Autodesk Fusion 360 part; units mm, degrees
(part 2 of 2)
  spline S7 degree 5 poles (3.1969, -8.4131) (3.199, -8.4065) (3.2031, -8.3933) (3.2093, -8.3736) (3.2174, -8.3472) (3.2273, -8.3143) (3.237, -8.2814) (3.2465, -8.2485) (3.2557, -8.2156) (3.2647, -8.1828) (3.2735, -8.1499) (3.282, -8.1171) (3.2903, -8.0843) (3.2983, -8.0515) (3.3062, -8.0188) (3.3138, -7.986) (3.3211, -7.9533) (3.3282, -7.9206) (3.3351, -7.888) (3.3418, -7.8554) (3.3482, -7.8228) (3.3543, -7.7902) (3.3602, -7.7577) (3.3659, -7.7253) (3.3713, -7.6928) (3.3765, -7.6604) (3.3814, -7.6281) (3.3861, -7.5958) (3.3906, -7.5635) (3.3947, -7.5313) (3.3987, -7.4991) (3.4023, -7.467) (3.4058, -7.4349) (3.4089, -7.4029) (3.4118, -7.371) (3.4145, -7.3391) (3.4169, -7.3073) (3.419, -7.2755) (3.4208, -7.2438) (3.4224, -7.2122) (3.4238, -7.1806) (3.4248, -7.1491) (3.4256, -7.1177) (3.426, -7.0864) (3.4262, -7.0551) (3.4262, -7.024) (3.4258, -6.9929) (3.4252, -6.9619) (3.4242, -6.931) (3.423, -6.9002) (3.4215, -6.8695) (3.4196, -6.8389) (3.4175, -6.8084) (3.415, -6.778) (3.4121, -6.7477) (3.409, -6.7176) (3.4055, -6.6876) (3.4018, -6.6576) (3.3978, -6.6278) (3.3934, -6.5981) (3.3886, -6.5686) (3.3833, -6.5393) (3.3775, -6.5102) (3.3713, -6.4813) (3.3645, -6.4526) (3.3575, -6.424) (3.3502, -6.3955) (3.3426, -6.3672) (3.3348, -6.339) (3.3263, -6.3112) (3.3168, -6.2838) (3.3081, -6.2623) (3.3008, -6.2466) (3.2955, -6.2363) (3.2928, -6.2312) knots -1 -1 -1 -1 -1 -1 -0.98571429 -0.97142857 -0.95714286 -0.94285714 -0.92857143 -0.91428571 -0.9 -0.88571429 -0.87142857 -0.85714286 -0.84285714 -0.82857143 -0.81428571 -0.8 -0.78571429 -0.77142857 -0.75714286 -0.74285714 -0.72857143 -0.71428571 -0.7 -0.68571429 -0.67142857 -0.65714286 -0.64285714 -0.62857143 -0.61428571 -0.6 -0.58571429 -0.57142857 -0.55714286 -0.54285714 -0.52857143 -0.51428571 -0.5 -0.48571429 -0.47142857 -0.45714286 -0.44285714 -0.42857143 -0.41428571 -0.4 -0.38571429 -0.37142857 -0.35714286 -0.34285714 -0.32857143 -0.31428571 -0.3 -0.28571429 -0.27142857 -0.25714286 -0.24285714 -0.22857143 -0.21428571 -0.2 -0.18571429 -0.17142857 -0.15714286 -0.14285714 -0.12857143 -0.11428571 -0.1 -0.08571429 -0.07142857 -0.05714286 -0.04285714 -0.02857143 -0.01428571 0 0 0 0 0 0
  line L7 (3.2928, -6.2312) -> (2.9176, -5.521)
  arc A15 (3.0915, -4.8654) -> (2.9176, -5.521) centre (3.3596, -5.2874) ccw
  arc A16 (3.0915, -4.8654) -> (3.672, -4.4437) centre (0, 0) ccw
  arc A17 (4.3492, -4.4809) -> (3.672, -4.4437) centre (3.9905, -4.8291) ccw
  line L8 (4.3492, -4.4809) -> (4.9086, -5.0572)
  spline S8 degree 5 poles (4.9086, -5.0572) (4.9127, -5.0613) (4.9209, -5.0695) (4.9336, -5.0813) (4.9513, -5.0962) (4.9744, -5.1137) (4.9983, -5.1304) (5.0226, -5.1466) (5.0473, -5.1625) (5.0721, -5.1783) (5.097, -5.1938) (5.1223, -5.2091) (5.1478, -5.224) (5.1737, -5.2385) (5.2, -5.2525) (5.2266, -5.2662) (5.2535, -5.2796) (5.2806, -5.2926) (5.3079, -5.3054) (5.3354, -5.318) (5.3631, -5.3303) (5.391, -5.3423) (5.4191, -5.3541) (5.4474, -5.3656) (5.476, -5.3768) (5.5047, -5.3878) (5.5336, -5.3984) (5.5627, -5.4089) (5.592, -5.4191) (5.6215, -5.429) (5.6511, -5.4387) (5.6809, -5.4482) (5.7108, -5.4574) (5.7409, -5.4664) (5.7712, -5.4751) (5.8016, -5.4836) (5.8322, -5.4919) (5.8629, -5.4999) (5.8938, -5.5077) (5.9248, -5.5153) (5.9559, -5.5226) (5.9872, -5.5297) (6.0186, -5.5366) (6.0501, -5.5433) (6.0818, -5.5497) (6.1136, -5.5559) (6.1456, -5.5619) (6.1776, -5.5676) (6.2098, -5.5731) (6.2421, -5.5784) (6.2745, -5.5835) (6.307, -5.5884) (6.3397, -5.593) (6.3724, -5.5975) (6.4053, -5.6017) (6.4383, -5.6056) (6.4713, -5.6094) (6.5045, -5.613) (6.5378, -5.6163) (6.5712, -5.6194) (6.6046, -5.6223) (6.6382, -5.625) (6.6719, -5.6274) (6.7056, -5.6297) (6.7395, -5.6317) (6.7734, -5.6335) (6.8075, -5.6351) (6.8416, -5.6365) (6.8758, -5.6377) (6.9101, -5.6386) (6.9444, -5.6394) (6.972, -5.6398) (6.9927, -5.64) (7.0065, -5.6401) (7.0134, -5.6402) knots 0 0 0 0 0 0 0.01428571 0.02857143 0.04285714 0.05714286 0.07142857 0.08571429 0.1 0.11428571 0.12857143 0.14285714 0.15714286 0.17142857 0.18571429 0.2 0.21428571 0.22857143 0.24285714 0.25714286 0.27142857 0.28571429 0.3 0.31428571 0.32857143 0.34285714 0.35714286 0.37142857 0.38571429 0.4 0.41428571 0.42857143 0.44285714 0.45714286 0.47142857 0.48571429 0.5 0.51428571 0.52857143 0.54285714 0.55714286 0.57142857 0.58571429 0.6 0.61428571 0.62857143 0.64285714 0.65714286 0.67142857 0.68571429 0.7 0.71428571 0.72857143 0.74285714 0.75714286 0.77142857 0.78571429 0.8 0.81428571 0.82857143 0.84285714 0.85714286 0.87142857 0.88571429 0.9 0.91428571 0.92857143 0.94285714 0.95714286 0.97142857 0.98571429 1 1 1 1 1 1
  arc A18 (7.0134, -5.6402) -> (7.5314, -4.9273) centre (0, 0) ccw
  spline S9 degree 5 poles (7.5314, -4.9273) (7.5292, -4.9207) (7.5249, -4.9076) (7.5182, -4.888) (7.5093, -4.8619) (7.498, -4.8294) (7.4865, -4.7971) (7.4748, -4.765) (7.4629, -4.7329) (7.4509, -4.7011) (7.4387, -4.6693) (7.4263, -4.6378) (7.4137, -4.6064) (7.401, -4.5751) (7.3881, -4.544) (7.375, -4.5131) (7.3617, -4.4823) (7.3482, -4.4516) (7.3346, -4.4212) (7.3208, -4.3909) (7.3068, -4.3608) (7.2927, -4.3308) (7.2784, -4.301) (7.2639, -4.2714) (7.2492, -4.242) (7.2343, -4.2127) (7.2193, -4.1837) (7.2041, -4.1548) (7.1887, -4.1261) (7.1732, -4.0976) (7.1574, -4.0692) (7.1415, -4.0411) (7.1255, -4.0131) (7.1092, -3.9854) (7.0928, -3.9578) (7.0762, -3.9305) (7.0594, -3.9033) (7.0425, -3.8764) (7.0253, -3.8496) (7.008, -3.8231) (6.9905, -3.7968) (6.9729, -3.7707) (6.955, -3.7449) (6.937, -3.7192) (6.9188, -3.6938) (6.9004, -3.6687) (6.8819, -3.6437) (6.8631, -3.619) (6.8442, -3.5946) (6.8251, -3.5704) (6.8058, -3.5464) (6.7863, -3.5227) (6.7667, -3.4993) (6.7468, -3.4763) (6.7267, -3.4534) (6.7064, -3.4309) (6.686, -3.4086) (6.6654, -3.3866) (6.6446, -3.3649) (6.6236, -3.3434) (6.6024, -3.3224) (6.5809, -3.3017) (6.5591, -3.2816) (6.537, -3.2619) (6.5147, -3.2426) (6.4922, -3.2236) (6.4695, -3.2049) (6.4468, -3.1864) (6.4239, -3.1683) (6.4006, -3.1507) (6.3768, -3.1341) (6.3572, -3.1219) (6.342, -3.1135) (6.3317, -3.1082) (6.3265, -3.1056) knots -1 -1 -1 -1 -1 -1 -0.98571429 -0.97142857 -0.95714286 -0.94285714 -0.92857143 -0.91428571 -0.9 -0.88571429 -0.87142857 -0.85714286 -0.84285714 -0.82857143 -0.81428571 -0.8 -0.78571429 -0.77142857 -0.75714286 -0.74285714 -0.72857143 -0.71428571 -0.7 -0.68571429 -0.67142857 -0.65714286 -0.64285714 -0.62857143 -0.61428571 -0.6 -0.58571429 -0.57142857 -0.55714286 -0.54285714 -0.52857143 -0.51428571 -0.5 -0.48571429 -0.47142857 -0.45714286 -0.44285714 -0.42857143 -0.41428571 -0.4 -0.38571429 -0.37142857 -0.35714286 -0.34285714 -0.32857143 -0.31428571 -0.3 -0.28571429 -0.27142857 -0.25714286 -0.24285714 -0.22857143 -0.21428571 -0.2 -0.18571429 -0.17142857 -0.15714286 -0.14285714 -0.12857143 -0.11428571 -0.1 -0.08571429 -0.07142857 -0.05714286 -0.04285714 -0.02857143 -0.01428571 0 0 0 0 0 0
  line L9 (6.3265, -3.1056) -> (5.6055, -2.7517)
  arc A19 (5.3609, -2.1191) -> (5.6055, -2.7517) centre (5.8259, -2.3029) ccw
  arc A20 (5.3609, -2.1191) -> (5.5826, -1.4367) centre (0, 0) ccw
  arc A21 (6.1524, -1.0687) -> (5.5826, -1.4367) centre (6.0668, -1.5613) ccw
  line L10 (6.1524, -1.0687) -> (6.9437, -1.2061)
  spline S10 degree 5 poles (6.9437, -1.2061) (6.9494, -1.2071) (6.9609, -1.2089) (6.9781, -1.211) (7.0011, -1.2127) (7.0301, -1.2132) (7.0593, -1.2127) (7.0885, -1.2115) (7.1178, -1.2099) (7.1471, -1.208) (7.1764, -1.2059) (7.2058, -1.2034) (7.2353, -1.2005) (7.2647, -1.197) (7.2943, -1.1929) (7.3238, -1.1884) (7.3534, -1.1833) (7.383, -1.178) (7.4126, -1.1723) (7.4422, -1.1663) (7.4719, -1.1599) (7.5015, -1.1533) (7.5312, -1.1463) (7.5609, -1.139) (7.5906, -1.1313) (7.6202, -1.1232) (7.6499, -1.1148) (7.6796, -1.1062) (7.7093, -1.0972) (7.7389, -1.0879) (7.7686, -1.0784) (7.7983, -1.0685) (7.8279, -1.0584) (7.8575, -1.048) (7.8872, -1.0372) (7.9168, -1.0262) (7.9464, -1.015) (7.9759, -1.0034) (8.0055, -0.9916) (8.035, -0.9795) (8.0645, -0.9671) (8.094, -0.9545) (8.1235, -0.9416) (8.1529, -0.9284) (8.1823, -0.915) (8.2117, -0.9013) (8.241, -0.8874) (8.2704, -0.8732) (8.2996, -0.8587) (8.3289, -0.844) (8.3581, -0.8291) (8.3873, -0.8139) (8.4164, -0.7985) (8.4455, -0.7828) (8.4746, -0.7669) (8.5036, -0.7508) (8.5325, -0.7344) (8.5615, -0.7177) (8.5903, -0.7009) (8.6192, -0.6838) (8.648, -0.6664) (8.6767, -0.6489) (8.7054, -0.6311) (8.734, -0.613) (8.7626, -0.5948) (8.7911, -0.5763) (8.8196, -0.5576) (8.848, -0.5387) (8.8764, -0.5195) (8.9047, -0.5001) (8.9329, -0.4805) (8.9555, -0.4647) (8.9723, -0.4527) (8.9836, -0.4446) (8.9892, -0.4406) knots 0 0 0 0 0 0 0.01428571 0.02857143 0.04285714 0.05714286 0.07142857 0.08571429 0.1 0.11428571 0.12857143 0.14285714 0.15714286 0.17142857 0.18571429 0.2 0.21428571 0.22857143 0.24285714 0.25714286 0.27142857 0.28571429 0.3 0.31428571 0.32857143 0.34285714 0.35714286 0.37142857 0.38571429 0.4 0.41428571 0.42857143 0.44285714 0.45714286 0.47142857 0.48571429 0.5 0.51428571 0.52857143 0.54285714 0.55714286 0.57142857 0.58571429 0.6 0.61428571 0.62857143 0.64285714 0.65714286 0.67142857 0.68571429 0.7 0.71428571 0.72857143 0.74285714 0.75714286 0.77142857 0.78571429 0.8 0.81428571 0.82857143 0.84285714 0.85714286 0.87142857 0.88571429 0.9 0.91428571 0.92857143 0.94285714 0.95714286 0.97142857 0.98571429 1 1 1 1 1 1
  arc A22 (8.9892, -0.4406) -> (8.9892, 0.4406) centre (0, 0) ccw
  spline S11 degree 5 poles (8.9892, 0.4406) (8.9836, 0.4446) (8.9723, 0.4527) (8.9555, 0.4647) (8.9329, 0.4805) (8.9047, 0.5001) (8.8764, 0.5195) (8.848, 0.5387) (8.8196, 0.5576) (8.7911, 0.5763) (8.7626, 0.5948) (8.734, 0.613) (8.7054, 0.6311) (8.6767, 0.6489) (8.648, 0.6664) (8.6192, 0.6838) (8.5903, 0.7009) (8.5615, 0.7177) (8.5325, 0.7344) (8.5036, 0.7508) (8.4746, 0.7669) (8.4455, 0.7828) (8.4164, 0.7985) (8.3873, 0.8139) (8.3581, 0.8291) (8.3289, 0.844) (8.2996, 0.8587) (8.2704, 0.8732) (8.241, 0.8874) (8.2117, 0.9013) (8.1823, 0.915) (8.1529, 0.9284) (8.1235, 0.9416) (8.094, 0.9545) (8.0645, 0.9671) (8.035, 0.9795) (8.0055, 0.9916) (7.9759, 1.0034) (7.9464, 1.015) (7.9168, 1.0262) (7.8872, 1.0372) (7.8575, 1.048) (7.8279, 1.0584) (7.7983, 1.0685) (7.7686, 1.0784) (7.7389, 1.0879) (7.7093, 1.0972) (7.6796, 1.1062) (7.6499, 1.1148) (7.6202, 1.1232) (7.5906, 1.1313) (7.5609, 1.139) (7.5312, 1.1463) (7.5015, 1.1533) (7.4719, 1.1599) (7.4422, 1.1663) (7.4126, 1.1723) (7.383, 1.178) (7.3534, 1.1833) (7.3238, 1.1884) (7.2943, 1.1929) (7.2647, 1.197) (7.2353, 1.2005) (7.2058, 1.2034) (7.1764, 1.2059) (7.1471, 1.208) (7.1178, 1.2099) (7.0885, 1.2115) (7.0593, 1.2127) (7.0301, 1.2132) (7.0011, 1.2127) (6.9781, 1.211) (6.9609, 1.2089) (6.9494, 1.2071) (6.9437, 1.2061) knots -1 -1 -1 -1 -1 -1 -0.98571429 -0.97142857 -0.95714286 -0.94285714 -0.92857143 -0.91428571 -0.9 -0.88571429 -0.87142857 -0.85714286 -0.84285714 -0.82857143 -0.81428571 -0.8 -0.78571429 -0.77142857 -0.75714286 -0.74285714 -0.72857143 -0.71428571 -0.7 -0.68571429 -0.67142857 -0.65714286 -0.64285714 -0.62857143 -0.61428571 -0.6 -0.58571429 -0.57142857 -0.55714286 -0.54285714 -0.52857143 -0.51428571 -0.5 -0.48571429 -0.47142857 -0.45714286 -0.44285714 -0.42857143 -0.41428571 -0.4 -0.38571429 -0.37142857 -0.35714286 -0.34285714 -0.32857143 -0.31428571 -0.3 -0.28571429 -0.27142857 -0.25714286 -0.24285714 -0.22857143 -0.21428571 -0.2 -0.18571429 -0.17142857 -0.15714286 -0.14285714 -0.12857143 -0.11428571 -0.1 -0.08571429 -0.07142857 -0.05714286 -0.04285714 -0.02857143 -0.01428571 0 0 0 0 0 0
  line L11 (6.9437, 1.2061) -> (6.1524, 1.0687)
  arc A23 (5.5826, 1.4367) -> (6.1524, 1.0687) centre (6.0668, 1.5613) ccw
  arc A24 (5.5826, 1.4367) -> (5.3609, 2.1191) centre (0, 0) ccw
  arc A25 (5.6055, 2.7517) -> (5.3609, 2.1191) centre (5.8259, 2.3029) ccw
  line L12 (5.6055, 2.7517) -> (6.3265, 3.1056)
  spline S12 degree 5 poles (6.3265, 3.1056) (6.3317, 3.1082) (6.342, 3.1135) (6.3572, 3.1219) (6.3768, 3.1341) (6.4006, 3.1507) (6.4239, 3.1683) (6.4468, 3.1864) (6.4695, 3.2049) (6.4922, 3.2236) (6.5147, 3.2426) (6.537, 3.2619) (6.5591, 3.2816) (6.5809, 3.3017) (6.6024, 3.3224) (6.6236, 3.3434) (6.6446, 3.3649) (6.6654, 3.3866) (6.686, 3.4086) (6.7064, 3.4309) (6.7267, 3.4534) (6.7468, 3.4763) (6.7667, 3.4993) (6.7863, 3.5227) (6.8058, 3.5464) (6.8251, 3.5704) (6.8442, 3.5946) (6.8631, 3.619) (6.8819, 3.6437) (6.9004, 3.6687) (6.9188, 3.6938) (6.937, 3.7192) (6.955, 3.7449) (6.9729, 3.7707) (6.9905, 3.7968) (7.008, 3.8231) (7.0253, 3.8496) (7.0425, 3.8764) (7.0594, 3.9033) (7.0762, 3.9305) (7.0928, 3.9578) (7.1092, 3.9854) (7.1255, 4.0131) (7.1415, 4.0411) (7.1574, 4.0692) (7.1732, 4.0976) (7.1887, 4.1261) (7.2041, 4.1548) (7.2193, 4.1837) (7.2343, 4.2127) (7.2492, 4.242) (7.2639, 4.2714) (7.2784, 4.301) (7.2927, 4.3308) (7.3068, 4.3608) (7.3208, 4.3909) (7.3346, 4.4212) (7.3482, 4.4516) (7.3617, 4.4823) (7.375, 4.5131) (7.3881, 4.544) (7.401, 4.5751) (7.4137, 4.6064) (7.4263, 4.6378) (7.4387, 4.6693) (7.4509, 4.7011) (7.4629, 4.7329) (7.4748, 4.765) (7.4865, 4.7971) (7.498, 4.8294) (7.5093, 4.8619) (7.5182, 4.888) (7.5249, 4.9076) (7.5292, 4.9207) (7.5314, 4.9273) knots 0 0 0 0 0 0 0.01428571 0.02857143 0.04285714 0.05714286 0.07142857 0.08571429 0.1 0.11428571 0.12857143 0.14285714 0.15714286 0.17142857 0.18571429 0.2 0.21428571 0.22857143 0.24285714 0.25714286 0.27142857 0.28571429 0.3 0.31428571 0.32857143 0.34285714 0.35714286 0.37142857 0.38571429 0.4 0.41428571 0.42857143 0.44285714 0.45714286 0.47142857 0.48571429 0.5 0.51428571 0.52857143 0.54285714 0.55714286 0.57142857 0.58571429 0.6 0.61428571 0.62857143 0.64285714 0.65714286 0.67142857 0.68571429 0.7 0.71428571 0.72857143 0.74285714 0.75714286 0.77142857 0.78571429 0.8 0.81428571 0.82857143 0.84285714 0.85714286 0.87142857 0.88571429 0.9 0.91428571 0.92857143 0.94285714 0.95714286 0.97142857 0.98571429 1 1 1 1 1 1
  arc A26 (7.5314, 4.9273) -> (7.0134, 5.6402) centre (0, 0) ccw
  spline S13 degree 5 poles (7.0134, 5.6402) (7.0065, 5.6401) (6.9927, 5.64) (6.972, 5.6398) (6.9444, 5.6394) (6.9101, 5.6386) (6.8758, 5.6377) (6.8416, 5.6365) (6.8075, 5.6351) (6.7734, 5.6335) (6.7395, 5.6317) (6.7056, 5.6297) (6.6719, 5.6274) (6.6382, 5.625) (6.6046, 5.6223) (6.5712, 5.6194) (6.5378, 5.6163) (6.5045, 5.613) (6.4713, 5.6094) (6.4383, 5.6056) (6.4053, 5.6017) (6.3724, 5.5975) (6.3397, 5.593) (6.307, 5.5884) (6.2745, 5.5835) (6.2421, 5.5784) (6.2098, 5.5731) (6.1776, 5.5676) (6.1456, 5.5619) (6.1136, 5.5559) (6.0818, 5.5497) (6.0501, 5.5433) (6.0186, 5.5366) (5.9872, 5.5297) (5.9559, 5.5226) (5.9248, 5.5153) (5.8938, 5.5077) (5.8629, 5.4999) (5.8322, 5.4919) (5.8016, 5.4836) (5.7712, 5.4751) (5.7409, 5.4664) (5.7108, 5.4574) (5.6809, 5.4482) (5.6511, 5.4387) (5.6215, 5.429) (5.592, 5.4191) (5.5627, 5.4089) (5.5336, 5.3984) (5.5047, 5.3878) (5.476, 5.3768) (5.4474, 5.3656) (5.4191, 5.3541) (5.391, 5.3423) (5.3631, 5.3303) (5.3354, 5.318) (5.3079, 5.3054) (5.2806, 5.2926) (5.2535, 5.2796) (5.2266, 5.2662) (5.2, 5.2525) (5.1737, 5.2385) (5.1478, 5.224) (5.1223, 5.2091) (5.097, 5.1938) (5.0721, 5.1783) (5.0473, 5.1625) (5.0226, 5.1466) (4.9983, 5.1304) (4.9744, 5.1137) (4.9513, 5.0962) (4.9336, 5.0813) (4.9209, 5.0695) (4.9127, 5.0613) (4.9086, 5.0572) knots -1 -1 -1 -1 -1 -1 -0.98571429 -0.97142857 -0.95714286 -0.94285714 -0.92857143 -0.91428571 -0.9 -0.88571429 -0.87142857 -0.85714286 -0.84285714 -0.82857143 -0.81428571 -0.8 -0.78571429 -0.77142857 -0.75714286 -0.74285714 -0.72857143 -0.71428571 -0.7 -0.68571429 -0.67142857 -0.65714286 -0.64285714 -0.62857143 -0.61428571 -0.6 -0.58571429 -0.57142857 -0.55714286 -0.54285714 -0.52857143 -0.51428571 -0.5 -0.48571429 -0.47142857 -0.45714286 -0.44285714 -0.42857143 -0.41428571 -0.4 -0.38571429 -0.37142857 -0.35714286 -0.34285714 -0.32857143 -0.31428571 -0.3 -0.28571429 -0.27142857 -0.25714286 -0.24285714 -0.22857143 -0.21428571 -0.2 -0.18571429 -0.17142857 -0.15714286 -0.14285714 -0.12857143 -0.11428571 -0.1 -0.08571429 -0.07142857 -0.05714286 -0.04285714 -0.02857143 -0.01428571 0 0 0 0 0 0
  line L13 (4.9086, 5.0572) -> (4.3492, 4.4809)
  arc A27 (3.672, 4.4437) -> (4.3492, 4.4809) centre (3.9905, 4.8291) ccw
  arc A28 (3.672, 4.4437) -> (3.0915, 4.8654) centre (0, 0) ccw
  arc A29 (2.9176, 5.521) -> (3.0915, 4.8654) centre (3.3596, 5.2874) ccw
  line L14 (2.9176, 5.521) -> (3.2928, 6.2312)
  spline S14 degree 5 poles (3.2928, 6.2312) (3.2955, 6.2363) (3.3008, 6.2466) (3.3081, 6.2623) (3.3168, 6.2838) (3.3263, 6.3112) (3.3348, 6.339) (3.3426, 6.3672) (3.3502, 6.3955) (3.3575, 6.424) (3.3645, 6.4526) (3.3713, 6.4813) (3.3775, 6.5102) (3.3833, 6.5393) (3.3886, 6.5686) (3.3934, 6.5981) (3.3978, 6.6278) (3.4018, 6.6576) (3.4055, 6.6876) (3.409, 6.7176) (3.4121, 6.7477) (3.415, 6.778) (3.4175, 6.8084) (3.4196, 6.8389) (3.4215, 6.8695) (3.423, 6.9002) (3.4242, 6.931) (3.4252, 6.9619) (3.4258, 6.9929) (3.4262, 7.024) (3.4262, 7.0551) (3.426, 7.0864) (3.4256, 7.1177) (3.4248, 7.1491) (3.4238, 7.1806) (3.4224, 7.2122) (3.4208, 7.2438) (3.419, 7.2755) (3.4169, 7.3073) (3.4145, 7.3391) (3.4118, 7.371) (3.4089, 7.4029) (3.4058, 7.4349) (3.4023, 7.467) (3.3987, 7.4991) (3.3947, 7.5313) (3.3906, 7.5635) (3.3861, 7.5958) (3.3814, 7.6281) (3.3765, 7.6604) (3.3713, 7.6928) (3.3659, 7.7253) (3.3602, 7.7577) (3.3543, 7.7902) (3.3482, 7.8228) (3.3418, 7.8554) (3.3351, 7.888) (3.3282, 7.9206) (3.3211, 7.9533) (3.3138, 7.986) (3.3062, 8.0188) (3.2983, 8.0515) (3.2903, 8.0843) (3.282, 8.1171) (3.2735, 8.1499) (3.2647, 8.1828) (3.2557, 8.2156) (3.2465, 8.2485) (3.237, 8.2814) (3.2273, 8.3143) (3.2174, 8.3472) (3.2093, 8.3736) (3.2031, 8.3933) (3.199, 8.4065) (3.1969, 8.4131) knots 0 0 0 0 0 0 0.01428571 0.02857143 0.04285714 0.05714286 0.07142857 0.08571429 0.1 0.11428571 0.12857143 0.14285714 0.15714286 0.17142857 0.18571429 0.2 0.21428571 0.22857143 0.24285714 0.25714286 0.27142857 0.28571429 0.3 0.31428571 0.32857143 0.34285714 0.35714286 0.37142857 0.38571429 0.4 0.41428571 0.42857143 0.44285714 0.45714286 0.47142857 0.48571429 0.5 0.51428571 0.52857143 0.54285714 0.55714286 0.57142857 0.58571429 0.6 0.61428571 0.62857143 0.64285714 0.65714286 0.67142857 0.68571429 0.7 0.71428571 0.72857143 0.74285714 0.75714286 0.77142857 0.78571429 0.8 0.81428571 0.82857143 0.84285714 0.85714286 0.87142857 0.88571429 0.9 0.91428571 0.92857143 0.94285714 0.95714286 0.97142857 0.98571429 1 1 1 1 1 1
  arc A30 (3.1969, 8.4131) -> (2.3588, 8.6854) centre (0, 0) ccw
  spline S15 degree 5 poles (2.3588, 8.6854) (2.3532, 8.6813) (2.3421, 8.6731) (2.3255, 8.6607) (2.3034, 8.6442) (2.276, 8.6234) (2.2489, 8.6025) (2.2219, 8.5814) (2.1951, 8.5602) (2.1685, 8.5389) (2.1421, 8.5175) (2.1159, 8.496) (2.0899, 8.4743) (2.0641, 8.4525) (2.0386, 8.4306) (2.0132, 8.4086) (1.988, 8.3865) (1.963, 8.3642) (1.9383, 8.3419) (1.9137, 8.3194) (1.8894, 8.2968) (1.8653, 8.2741) (1.8414, 8.2512) (1.8177, 8.2283) (1.7943, 8.2052) (1.771, 8.1821) (1.748, 8.1588) (1.7252, 8.1354) (1.7027, 8.1119) (1.6804, 8.0883) (1.6583, 8.0646) (1.6364, 8.0408) (1.6148, 8.0168) (1.5934, 7.9928) (1.5723, 7.9687) (1.5514, 7.9444) (1.5308, 7.9201) (1.5104, 7.8956) (1.4903, 7.8711) (1.4704, 7.8464) (1.4508, 7.8217) (1.4314, 7.7968) (1.4124, 7.7719) (1.3936, 7.7468) (1.375, 7.7216) (1.3568, 7.6964) (1.3388, 7.671) (1.3211, 7.6456) (1.3037, 7.62) (1.2865, 7.5944) (1.2697, 7.5686) (1.2532, 7.5428) (1.2371, 7.5168) (1.2212, 7.4908) (1.2058, 7.4646) (1.1906, 7.4384) (1.1757, 7.4121) (1.1611, 7.3857) (1.1469, 7.3592) (1.133, 7.3326) (1.1195, 7.3059) (1.1065, 7.2791) (1.0941, 7.2521) (1.0822, 7.225) (1.0708, 7.1978) (1.0597, 7.1706) (1.0489, 7.1433) (1.0383, 7.1159) (1.0281, 7.0885) (1.0186, 7.061) (1.0102, 7.0332) (1.0046, 7.0108) (1.0013, 6.9937) (0.9995, 6.9823) (0.9986, 6.9766) knots -1 -1 -1 -1 -1 -1 -0.98571429 -0.97142857 -0.95714286 -0.94285714 -0.92857143 -0.91428571 -0.9 -0.88571429 -0.87142857 -0.85714286 -0.84285714 -0.82857143 -0.81428571 -0.8 -0.78571429 -0.77142857 -0.75714286 -0.74285714 -0.72857143 -0.71428571 -0.7 -0.68571429 -0.67142857 -0.65714286 -0.64285714 -0.62857143 -0.61428571 -0.6 -0.58571429 -0.57142857 -0.55714286 -0.54285714 -0.52857143 -0.51428571 -0.5 -0.48571429 -0.47142857 -0.45714286 -0.44285714 -0.42857143 -0.41428571 -0.4 -0.38571429 -0.37142857 -0.35714286 -0.34285714 -0.32857143 -0.31428571 -0.3 -0.28571429 -0.27142857 -0.25714286 -0.24285714 -0.22857143 -0.21428571 -0.2 -0.18571429 -0.17142857 -0.15714286 -0.14285714 -0.12857143 -0.11428571 -0.1 -0.08571429 -0.07142857 -0.05714286 -0.04285714 -0.02857143 -0.01428571 0 0 0 0 0 0
  line L15 (0.9986, 6.9766) -> (0.8848, 6.1815)
  arc A31 (0.3588, 5.7533) -> (0.8848, 6.1815) centre (0.3899, 6.2524) ccw
  arc A32 (0.3588, 5.7533) -> (-0.3588, 5.7533) centre (0, 0) ccw
  arc A33 (-0.8848, 6.1815) -> (-0.3588, 5.7533) centre (-0.3899, 6.2524) ccw
  line L16 (-0.8848, 6.1815) -> (-0.9986, 6.9766)
  spline S16 degree 5 poles (-0.9986, 6.9766) (-0.9995, 6.9823) (-1.0013, 6.9937) (-1.0046, 7.0108) (-1.0102, 7.0332) (-1.0186, 7.061) (-1.0281, 7.0885) (-1.0383, 7.1159) (-1.0489, 7.1433) (-1.0597, 7.1706) (-1.0708, 7.1978) (-1.0822, 7.225) (-1.0941, 7.2521) (-1.1065, 7.2791) (-1.1195, 7.3059) (-1.133, 7.3326) (-1.1469, 7.3592) (-1.1611, 7.3857) (-1.1757, 7.4121) (-1.1906, 7.4384) (-1.2058, 7.4646) (-1.2212, 7.4908) (-1.2371, 7.5168) (-1.2532, 7.5428) (-1.2697, 7.5686) (-1.2865, 7.5944) (-1.3037, 7.62) (-1.3211, 7.6456) (-1.3388, 7.671) (-1.3568, 7.6964) (-1.375, 7.7216) (-1.3936, 7.7468) (-1.4124, 7.7719) (-1.4314, 7.7968) (-1.4508, 7.8217) (-1.4704, 7.8464) (-1.4903, 7.8711) (-1.5104, 7.8956) (-1.5308, 7.9201) (-1.5514, 7.9444) (-1.5723, 7.9687) (-1.5934, 7.9928) (-1.6148, 8.0168) (-1.6364, 8.0408) (-1.6583, 8.0646) (-1.6804, 8.0883) (-1.7027, 8.1119) (-1.7252, 8.1354) (-1.748, 8.1588) (-1.771, 8.1821) (-1.7943, 8.2052) (-1.8177, 8.2283) (-1.8414, 8.2512) (-1.8653, 8.2741) (-1.8894, 8.2968) (-1.9137, 8.3194) (-1.9383, 8.3419) (-1.963, 8.3642) (-1.988, 8.3865) (-2.0132, 8.4086) (-2.0386, 8.4306) (-2.0641, 8.4525) (-2.0899, 8.4743) (-2.1159, 8.496) (-2.1421, 8.5175) (-2.1685, 8.5389) (-2.1951, 8.5602) (-2.2219, 8.5814) (-2.2489, 8.6025) (-2.276, 8.6234) (-2.3034, 8.6442) (-2.3255, 8.6607) (-2.3421, 8.6731) (-2.3532, 8.6813) (-2.3588, 8.6854) knots 0 0 0 0 0 0 0.01428571 0.02857143 0.04285714 0.05714286 0.07142857 0.08571429 0.1 0.11428571 0.12857143 0.14285714 0.15714286 0.17142857 0.18571429 0.2 0.21428571 0.22857143 0.24285714 0.25714286 0.27142857 0.28571429 0.3 0.31428571 0.32857143 0.34285714 0.35714286 0.37142857 0.38571429 0.4 0.41428571 0.42857143 0.44285714 0.45714286 0.47142857 0.48571429 0.5 0.51428571 0.52857143 0.54285714 0.55714286 0.57142857 0.58571429 0.6 0.61428571 0.62857143 0.64285714 0.65714286 0.67142857 0.68571429 0.7 0.71428571 0.72857143 0.74285714 0.75714286 0.77142857 0.78571429 0.8 0.81428571 0.82857143 0.84285714 0.85714286 0.87142857 0.88571429 0.9 0.91428571 0.92857143 0.94285714 0.95714286 0.97142857 0.98571429 1 1 1 1 1 1
  arc A34 (-2.3588, 8.6854) -> (-3.1969, 8.4131) centre (0, 0) ccw
  spline S17 degree 5 poles (-3.1969, 8.4131) (-3.199, 8.4065) (-3.2031, 8.3933) (-3.2093, 8.3736) (-3.2174, 8.3472) (-3.2273, 8.3143) (-3.237, 8.2814) (-3.2465, 8.2485) (-3.2557, 8.2156) (-3.2647, 8.1828) (-3.2735, 8.1499) (-3.282, 8.1171) (-3.2903, 8.0843) (-3.2983, 8.0515) (-3.3062, 8.0188) (-3.3138, 7.986) (-3.3211, 7.9533) (-3.3282, 7.9206) (-3.3351, 7.888) (-3.3418, 7.8554) (-3.3482, 7.8228) (-3.3543, 7.7902) (-3.3602, 7.7577) (-3.3659, 7.7253) (-3.3713, 7.6928) (-3.3765, 7.6604) (-3.3814, 7.6281) (-3.3861, 7.5958) (-3.3906, 7.5635) (-3.3947, 7.5313) (-3.3987, 7.4991) (-3.4023, 7.467) (-3.4058, 7.4349) (-3.4089, 7.4029) (-3.4118, 7.371) (-3.4145, 7.3391) (-3.4169, 7.3073) (-3.419, 7.2755) (-3.4208, 7.2438) (-3.4224, 7.2122) (-3.4238, 7.1806) (-3.4248, 7.1491) (-3.4256, 7.1177) (-3.426, 7.0864) (-3.4262, 7.0551) (-3.4262, 7.024) (-3.4258, 6.9929) (-3.4252, 6.9619) (-3.4242, 6.931) (-3.423, 6.9002) (-3.4215, 6.8695) (-3.4196, 6.8389) (-3.4175, 6.8084) (-3.415, 6.778) (-3.4121, 6.7477) (-3.409, 6.7176) (-3.4055, 6.6876) (-3.4018, 6.6576) (-3.3978, 6.6278) (-3.3934, 6.5981) (-3.3886, 6.5686) (-3.3833, 6.5393) (-3.3775, 6.5102) (-3.3713, 6.4813) (-3.3645, 6.4526) (-3.3575, 6.424) (-3.3502, 6.3955) (-3.3426, 6.3672) (-3.3348, 6.339) (-3.3263, 6.3112) (-3.3168, 6.2838) (-3.3081, 6.2623) (-3.3008, 6.2466) (-3.2955, 6.2363) (-3.2928, 6.2312) knots -1 -1 -1 -1 -1 -1 -0.98571429 -0.97142857 -0.95714286 -0.94285714 -0.92857143 -0.91428571 -0.9 -0.88571429 -0.87142857 -0.85714286 -0.84285714 -0.82857143 -0.81428571 -0.8 -0.78571429 -0.77142857 -0.75714286 -0.74285714 -0.72857143 -0.71428571 -0.7 -0.68571429 -0.67142857 -0.65714286 -0.64285714 -0.62857143 -0.61428571 -0.6 -0.58571429 -0.57142857 -0.55714286 -0.54285714 -0.52857143 -0.51428571 -0.5 -0.48571429 -0.47142857 -0.45714286 -0.44285714 -0.42857143 -0.41428571 -0.4 -0.38571429 -0.37142857 -0.35714286 -0.34285714 -0.32857143 -0.31428571 -0.3 -0.28571429 -0.27142857 -0.25714286 -0.24285714 -0.22857143 -0.21428571 -0.2 -0.18571429 -0.17142857 -0.15714286 -0.14285714 -0.12857143 -0.11428571 -0.1 -0.08571429 -0.07142857 -0.05714286 -0.04285714 -0.02857143 -0.01428571 0 0 0 0 0 0
  line L17 (-3.2928, 6.2312) -> (-2.9176, 5.521)
  arc A35 (-3.0915, 4.8654) -> (-2.9176, 5.521) centre (-3.3596, 5.2874) ccw
  arc A36 (-3.0915, 4.8654) -> (-3.672, 4.4437) centre (0, 0) ccw
  arc A37 (-4.3492, 4.4809) -> (-3.672, 4.4437) centre (-3.9905, 4.8291) ccw
  line L18 (-4.3492, 4.4809) -> (-4.9086, 5.0572)
  spline S18 degree 5 poles (-4.9086, 5.0572) (-4.9127, 5.0613) (-4.9209, 5.0695) (-4.9336, 5.0813) (-4.9513, 5.0962) (-4.9744, 5.1137) (-4.9983, 5.1304) (-5.0226, 5.1466) (-5.0473, 5.1625) (-5.0721, 5.1783) (-5.097, 5.1938) (-5.1223, 5.2091) (-5.1478, 5.224) (-5.1737, 5.2385) (-5.2, 5.2525) (-5.2266, 5.2662) (-5.2535, 5.2796) (-5.2806, 5.2926) (-5.3079, 5.3054) (-5.3354, 5.318) (-5.3631, 5.3303) (-5.391, 5.3423) (-5.4191, 5.3541) (-5.4474, 5.3656) (-5.476, 5.3768) (-5.5047, 5.3878) (-5.5336, 5.3984) (-5.5627, 5.4089) (-5.592, 5.4191) (-5.6215, 5.429) (-5.6511, 5.4387) (-5.6809, 5.4482) (-5.7108, 5.4574) (-5.7409, 5.4664) (-5.7712, 5.4751) (-5.8016, 5.4836) (-5.8322, 5.4919) (-5.8629, 5.4999) (-5.8938, 5.5077) (-5.9248, 5.5153) (-5.9559, 5.5226) (-5.9872, 5.5297) (-6.0186, 5.5366) (-6.0501, 5.5433) (-6.0818, 5.5497) (-6.1136, 5.5559) (-6.1456, 5.5619) (-6.1776, 5.5676) (-6.2098, 5.5731) (-6.2421, 5.5784) (-6.2745, 5.5835) (-6.307, 5.5884) (-6.3397, 5.593) (-6.3724, 5.5975) (-6.4053, 5.6017) (-6.4383, 5.6056) (-6.4713, 5.6094) (-6.5045, 5.613) (-6.5378, 5.6163) (-6.5712, 5.6194) (-6.6046, 5.6223) (-6.6382, 5.625) (-6.6719, 5.6274) (-6.7056, 5.6297) (-6.7395, 5.6317) (-6.7734, 5.6335) (-6.8075, 5.6351) (-6.8416, 5.6365) (-6.8758, 5.6377) (-6.9101, 5.6386) (-6.9444, 5.6394) (-6.972, 5.6398) (-6.9927, 5.64) (-7.0065, 5.6401) (-7.0134, 5.6402) knots 0 0 0 0 0 0 0.01428571 0.02857143 0.04285714 0.05714286 0.07142857 0.08571429 0.1 0.11428571 0.12857143 0.14285714 0.15714286 0.17142857 0.18571429 0.2 0.21428571 0.22857143 0.24285714 0.25714286 0.27142857 0.28571429 0.3 0.31428571 0.32857143 0.34285714 0.35714286 0.37142857 0.38571429 0.4 0.41428571 0.42857143 0.44285714 0.45714286 0.47142857 0.48571429 0.5 0.51428571 0.52857143 0.54285714 0.55714286 0.57142857 0.58571429 0.6 0.61428571 0.62857143 0.64285714 0.65714286 0.67142857 0.68571429 0.7 0.71428571 0.72857143 0.74285714 0.75714286 0.77142857 0.78571429 0.8 0.81428571 0.82857143 0.84285714 0.85714286 0.87142857 0.88571429 0.9 0.91428571 0.92857143 0.94285714 0.95714286 0.97142857 0.98571429 1 1 1 1 1 1
  arc A38 (-7.0134, 5.6402) -> (-7.5314, 4.9273) centre (0, 0) ccw
  spline S19 degree 5 poles (-7.5314, 4.9273) (-7.5292, 4.9207) (-7.5249, 4.9076) (-7.5182, 4.888) (-7.5093, 4.8619) (-7.498, 4.8294) (-7.4865, 4.7971) (-7.4748, 4.765) (-7.4629, 4.7329) (-7.4509, 4.7011) (-7.4387, 4.6693) (-7.4263, 4.6378) (-7.4137, 4.6064) (-7.401, 4.5751) (-7.3881, 4.544) (-7.375, 4.5131) (-7.3617, 4.4823) (-7.3482, 4.4516) (-7.3346, 4.4212) (-7.3208, 4.3909) (-7.3068, 4.3608) (-7.2927, 4.3308) (-7.2784, 4.301) (-7.2639, 4.2714) (-7.2492, 4.242) (-7.2343, 4.2127) (-7.2193, 4.1837) (-7.2041, 4.1548) (-7.1887, 4.1261) (-7.1732, 4.0976) (-7.1574, 4.0692) (-7.1415, 4.0411) (-7.1255, 4.0131) (-7.1092, 3.9854) (-7.0928, 3.9578) (-7.0762, 3.9305) (-7.0594, 3.9033) (-7.0425, 3.8764) (-7.0253, 3.8496) (-7.008, 3.8231) (-6.9905, 3.7968) (-6.9729, 3.7707) (-6.955, 3.7449) (-6.937, 3.7192) (-6.9188, 3.6938) (-6.9004, 3.6687) (-6.8819, 3.6437) (-6.8631, 3.619) (-6.8442, 3.5946) (-6.8251, 3.5704) (-6.8058, 3.5464) (-6.7863, 3.5227) (-6.7667, 3.4993) (-6.7468, 3.4763) (-6.7267, 3.4534) (-6.7064, 3.4309) (-6.686, 3.4086) (-6.6654, 3.3866) (-6.6446, 3.3649) (-6.6236, 3.3434) (-6.6024, 3.3224) (-6.5809, 3.3017) (-6.5591, 3.2816) (-6.537, 3.2619) (-6.5147, 3.2426) (-6.4922, 3.2236) (-6.4695, 3.2049) (-6.4468, 3.1864) (-6.4239, 3.1683) (-6.4006, 3.1507) (-6.3768, 3.1341) (-6.3572, 3.1219) (-6.342, 3.1135) (-6.3317, 3.1082) (-6.3265, 3.1056) knots -1 -1 -1 -1 -1 -1 -0.98571429 -0.97142857 -0.95714286 -0.94285714 -0.92857143 -0.91428571 -0.9 -0.88571429 -0.87142857 -0.85714286 -0.84285714 -0.82857143 -0.81428571 -0.8 -0.78571429 -0.77142857 -0.75714286 -0.74285714 -0.72857143 -0.71428571 -0.7 -0.68571429 -0.67142857 -0.65714286 -0.64285714 -0.62857143 -0.61428571 -0.6 -0.58571429 -0.57142857 -0.55714286 -0.54285714 -0.52857143 -0.51428571 -0.5 -0.48571429 -0.47142857 -0.45714286 -0.44285714 -0.42857143 -0.41428571 -0.4 -0.38571429 -0.37142857 -0.35714286 -0.34285714 -0.32857143 -0.31428571 -0.3 -0.28571429 -0.27142857 -0.25714286 -0.24285714 -0.22857143 -0.21428571 -0.2 -0.18571429 -0.17142857 -0.15714286 -0.14285714 -0.12857143 -0.11428571 -0.1 -0.08571429 -0.07142857 -0.05714286 -0.04285714 -0.02857143 -0.01428571 0 0 0 0 0 0
  line L19 (-6.3265, 3.1056) -> (-5.6055, 2.7517)
  arc A39 (-5.3609, 2.1191) -> (-5.6055, 2.7517) centre (-5.8259, 2.3029) ccw
  line L20 (2.125, -1.9734) -> (-2.125, -1.9734)
  circle A40 centre (0, 0) radius 2.9
  line L21 (2.125, 1.9734) -> (-2.125, 1.9734)
  line L22 (-28.475, -1.7455) -> (-32.725, -1.7455)
  circle A41 centre (-30.6, 0) radius 2.75
  line L23 (-28.475, 1.7455) -> (-32.725, 1.7455)
  point P0 (-30.6, 0)
  point P1 (-30.6, 0)
  point P2 (-30.6, 0)
  point P3 (-30.6, 0)
  dimension "d17" = 5.8
  dimension "d18" = 4.25
  dimension "d19" = 5.5
  dimension "d20" = 4.25
  constraint coincident A0.centre A2.centre
  constraint coincident L20.start A40
  constraint coincident L20.end A40
  constraint horizontal L20
  constraint coincident L21.start A40
  constraint coincident L21.end A40
  constraint parallel L20 L21
  constraint equal L20 L21
  constraint coincident P3 P2
  constraint coincident L22.start A41
  constraint coincident L22.end A41
  constraint horizontal L22
  constraint coincident L23.start A41
  constraint coincident L23.end A41
  constraint parallel L22 L23
  constraint equal L22 L23
  measures "d17" diameter of A40
  measures "d18" distance of L20.start L20.end
  measures "d19" diameter of A41
  measures "d20" distance of L22.start L22.end
extrude "Extrude5" cut sketch "Sketch7" against normal up to surface (7 mm away) contours L20 A40 L21 bodies 1
extrude "Extrude6" add sketch "Sketch7" along normal blind 20 contours L22 A41 L23 bodies 2
named bodies: "Spur Gear (10 teeth)", "Spur Gear (30 teeth)"
